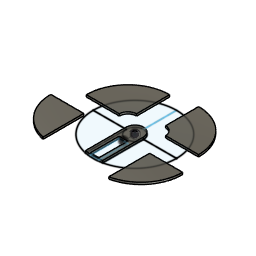
Lid Archive (Autodesk Fusion 360 design; units mm, degrees)
Autodesk Fusion 360 part; units mm, degrees
sketch "Lid" plane through (0, 0, 0) normal (0, 0, 1) x (1, 0, 0)
  circle A0 centre (0, 0) radius 145
  line L0 (0, 0) -> (0, -40) construction
  line L1 (-15, -40) -> (15, -40)
  line L2 (15, -40) -> (15, -140)
  line L3 (15, -140) -> (-15, -140)
  line L4 (-15, -140) -> (-15, -40)
  line L5 (0, 0) -> (2.5, 0) construction
  line L6 (0.845, -2.6554) -> (-2.6905, 0.8801)
  line L7 (-2.6905, 0.8801) -> (-0.9227, 2.6479)
  line L8 (-0.9227, 2.6479) -> (2.6128, -0.8876)
  line L9 (2.6128, -0.8876) -> (0.845, -2.6554)
  line L10 (-2.6905, 0.8801) -> (2.6128, -0.8876) construction
  line L11 (0.845, -2.6554) -> (-0.9227, 2.6479) construction
  circle A1 centre (0, 0) radius 30 construction
  line L12 (-30, 0) -> (-30, -141.8626) construction
  line L13 (30, 0) -> (30, -141.8626) construction
  line L14 (30, 0) -> (145, 0) construction
  line L15 (-30, 0) -> (-145, 0) construction
  line L16 (0.0657, 145) -> (0.0657, 29.9999) construction
  circle A2 centre (0, 0) radius 30
  line L17 (-30, 0) -> (-30, -141.8626)
  line L18 (30, 0) -> (30, -141.8626)
  line L19 (30, 0) -> (145, 0)
  line L20 (-30, 0) -> (-145, 0)
  line L21 (0.0657, 145) -> (0.0657, 29.9999)
  dimension "d17" = 290
  dimension "d18" = 40
  dimension "d19" = 30
  dimension "d20" = 100
  dimension "d29" = 5
  dimension "d30" = 2.5
  dimension "d40" = 60
  constraint coincident A0.centre L0.start
  constraint vertical L0
  constraint horizontal L1
  constraint vertical L2
  constraint horizontal L3
  constraint vertical L4
  constraint horizontal L5
  constraint concentric A0 A1
  constraint coincident A1 L12.start
  constraint coincident A0 L12.end
  constraint tangent A1 L12
  constraint parallel L0 L12
  constraint coincident A1 L13.start
  constraint coincident A0 L13.end
  constraint tangent A1 L13
  constraint vertical L13
  constraint coincident A0 L14.end
  constraint perpendicular L13 L14
  constraint coincident A0 L15.end
  constraint perpendicular L12 L15
  constraint coincident A0 L16.start
  constraint coincident A1 L16.end
  constraint vertical L16
  constraint tangent A2 L17
  measures "d17" diameter of A0
  measures "d18" distance of A0.centre L0.end
  measures "d19" distance of L1.start L1.end
  measures "d20" distance of L1.start L3.end
  measures "d29" distance of L6.start L6.end
  measures "d30" distance of L6.start L8.end
  measures "d40" diameter of A1
extrude "Extrude5" add sketch "Lid" along normal blind 7 contours A0 A2 L19 L21 makes body 1
move_body "Move1" bodies 1 to x (1, 0, 0) y (0, 1, 0) z (0, 0, 1) at (34.3045, 42.6002, 0)
extrude "Extrude6" add sketch "Lid" along normal blind 7 separate body contours A0 A2 L20 L21 makes body 2
move_body "Move2" bodies 2 to x (1, 0, 0) y (0, 1, 0) z (0, 0, 1) at (-52.0675, 28.0363, 0)
extrude "Extrude7" add sketch "Lid" along normal blind 7 separate body contours A0 L18 L19 makes body 3
move_body "Move3" bodies 3 to x (1, 0, 0) y (0, 1, 0) z (0, 0, 1) at (59.6328, -38.2718, 0)
extrude "Extrude8" add sketch "Lid" along normal blind 7 separate body contours A0 L17 L20 makes body 4
move_body "Move4" bodies 4 to x (1, 0, 0) y (0, 1, 0) z (0, 0, 1) at (-114.8154, -32.9316, 0)
extrude "Extrude9" add sketch "Lid" along normal blind 3 separate body contours L6 L7 L8 L9 makes body 5
extrude "Extrude10" add sketch "Lid" along normal blind 7 contours A0 A2 L17 L18 | A2 bodies 5
copy_body "Body->Comp1" bodies 5 removing the originals makes body 6 in component "Centre"
component "Centre" placed x (1, 0, 0) y (0, 1, 0) z (0, 0, 1) at (0, 0, 0)
named bodies: "Disc1", "Disc2", "Disc3", "Disc4", "Centre"
